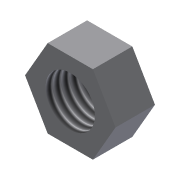
# Autodesk Inventor part: 3mm nut
Saved by Autodesk Inventor 2016 (Build 200138000, 138)
## iProperties
Created: 2014-11-22
Part Number: 3mm nut
Material: Generic
Document SubType Name: Modeling
Designer: Sebastian
Density: 1 g/cm^3
Appearance: Default
Mass: 0.0301905 g
Surface Area: 0.873782 cm^2
Volume: 0.0301905 cm^3
Author: Sebastian
Autodesk Inventor part; units mm, degrees
ref_plane "YZ Plane" through (0, 0, 0) normal (1, 0, 0) x (0, 1, 0)
ref_plane "XZ Plane" through (0, 0, 0) normal (0, 1, 0) x (-1, 0, 0)
ref_plane "XY Plane" through (0, 0, 0) normal (0, 0, 1) x (1, 0, 0)
sketch "Sketch1" plane through (0, 0, 0) normal (0, 1, 0) x (-1, 0, 0)
  line L0 (2.75, 0) -> (1.375, -2.3816)
  line L1 (1.375, -2.3816) -> (-1.375, -2.3816)
  line L2 (-1.375, -2.3816) -> (-2.75, 0)
  line L3 (-2.75, 0) -> (-1.375, 2.3816)
  line L4 (1.375, 2.3816) -> (2.75, 0)
  line L5 (1.375, 2.3816) -> (-1.375, 2.3816)
  circle A0 centre (0, 0) radius 1.5
  dimension "d19" = 3
  constraints: 12 end point, 2 parallel, 1 centre point, 1 coincident, 1 horizontal
  measures "d19" diameter of A0
extrude "Extrusion1" add sketch "Sketch1" along normal blind 2.4
thread "Thread1" size "M3x0.5" class "6H" standard "ANSI Metric M Profile" full length
body "Solid1"
